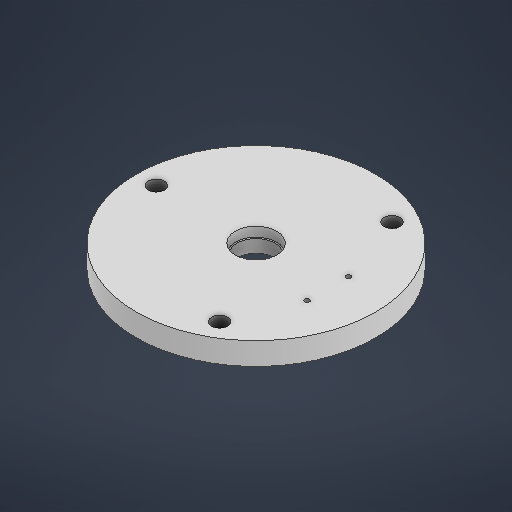
# Autodesk Inventor part: 1.1.1.Base Sta.Plate
Saved by Autodesk Inventor 2026.1 (Build 301233020, 233B)
## iProperties
Created: 2025-10-08
Part Number: 1.1.1.Base Sta.Plate
Material: Genérico
Document SubType Name: Modeling
Designer: vitos
Density: 1 g/cm^3
Appearance: Valor por defecto
Author: vitos
Autodesk Inventor part; units mm, degrees
ref_plane "YZ Plane" through (0, 0, 0) normal (1, 0, 0) x (0, 1, 0)
ref_plane "XZ Plane" through (0, 0, 0) normal (0, 1, 0) x (-1, 0, 0)
ref_plane "XY Plane" through (0, 0, 0) normal (0, 0, 1) x (1, 0, 0)
sketch "Boceto1" plane through (0, 0, 0) normal (0, 1, 0) x (-1, 0, 0)
  circle A0 centre (0, 0) radius 75
  circle A1 centre (0, 0) radius 62.5
  circle A2 centre (62.5, 0) radius 5
  circle A3 centre (0, 0) radius 13
  circle A4 centre (0, 0) radius 12
  circle A5 centre (-47.25, 15.2) radius 1.5
  circle A6 centre (-47.25, -10.8) radius 1.5
  circle A7 centre (-31.25, 54.1266) radius 5
  circle A8 centre (-31.25, -54.1266) radius 5
  constraints: 9 centre point, 4 coincident, 2 point on circle
extrude "Extrusión1" add sketch "Boceto1" along normal blind 14 contours A0 | A2 A1 A8 A7
extrude "Extrusión2" add sketch "Boceto1" along normal blind 8 contours A3
thread "Rosca1" size "M10x1.5" class "6H" standard "ANSI Metric M Profile" full length
thread "Rosca2" size "M10x1.5" class "6H" standard "ANSI Metric M Profile" full length
thread "Rosca3" size "M10x1.5" class "6H" standard "ANSI Metric M Profile" full length
thread "Rosca4" size "M3x0.5" class "6H" standard "ANSI Metric M Profile" full length
thread "Rosca5" size "M3x0.5" class "6H" standard "ANSI Metric M Profile" full length
